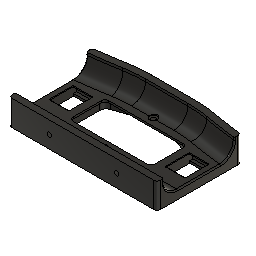
Filtered Mains Braket (Autodesk Fusion 360 design; units mm, degrees)
Autodesk Fusion 360 part; units mm, degrees
sketch "Mains Cutout" plane through (0, 0, 0) normal (0, 0, 1) x (1, 0, 0)
  line L0 (0, 25.5) -> (0, -25.5) construction
  line L1 (-33.15, 14.516) -> (33.15, -14.516) construction
  line L2 (33.15, 14.516) -> (-33.15, -14.516) construction
  line L3 (-33.15, 14.516) -> (33.15, 14.516) construction
  line L4 (33.15, 14.516) -> (33.15, -14.516) construction
  line L5 (33.15, -14.516) -> (-33.15, -14.516) construction
  line L6 (-33.15, -10.9343) -> (-33.15, 14.516) construction
  line L7 (29.7587, -15.6684) -> (1.6087, -25.2341)
  line L8 (-29.7587, -15.6684) -> (-1.6087, -25.2341)
  line L9 (-29.7587, 15.6684) -> (-1.6087, 25.2341)
  line L10 (29.7587, 15.6684) -> (1.6087, 25.2341)
  arc A0 (1.6087, 25.2341) -> (-1.6087, 25.2341) centre (0, 20.5) ccw
  arc A1 (-1.6087, -25.2341) -> (1.6087, -25.2341) centre (0, -20.5) ccw
  line L11 (33.15, 10.9343) -> (33.15, -10.9343) construction
  line L12 (-33.15, -14.516) -> (-33.15, 10.9343) construction
  circle A2 centre (0, 20) radius 1.65
  circle A3 centre (0, -20) radius 1.65
  line L13 (0, 20) -> (0, -20) construction
  circle A4 centre (0, 20) radius 3
  circle A5 centre (0, -20) radius 3
  line L14 (-29.2, 14.1) -> (29.2, 14.1)
  line L15 (32.2, 11.1) -> (32.2, -11.1)
  line L16 (29.2, -14.1) -> (-29.2, -14.1)
  line L17 (-32.2, -11.1) -> (-32.2, 11.1)
  arc A6 (32.2, 11.1) -> (29.2, 14.1) centre (29.2, 11.1) ccw
  arc A7 (29.2, -14.1) -> (32.2, -11.1) centre (29.2, -11.1) ccw
  arc A8 (-32.2, -11.1) -> (-29.2, -14.1) centre (-29.2, -11.1) ccw
  line L18 (29.2, 14.1) -> (32.2, 14.1) construction
  line L19 (32.2, 11.1) -> (32.2, 14.1) construction
  line L20 (32.2, -11.1) -> (32.2, -14.1) construction
  line L21 (29.2, -14.1) -> (32.2, -14.1) construction
  line L22 (-29.2, -14.1) -> (-32.2, -14.1) construction
  line L23 (-32.2, -11.1) -> (-32.2, -14.1) construction
  arc A9 (-29.2, 14.1) -> (-32.2, 11.1) centre (-29.2, 11.1) ccw
  line L24 (-29.2, 14.1) -> (-32.2, 14.1) construction
  line L25 (-32.2, 11.1) -> (-32.2, 14.1) construction
  arc A10 (-29.7587, 15.6684) -> (-33.15, 10.9343) centre (-28.15, 10.9343) ccw
  line L26 (-29.7587, 15.6684) -> (-33.15, 14.516) construction
  arc A11 (-33.15, -10.9343) -> (-29.7587, -15.6684) centre (-28.15, -10.9343) ccw
  line L27 (-29.7587, -15.6684) -> (-33.15, -14.516) construction
  line L28 (-33.15, 10.9343) -> (-33.15, -10.9343)
  arc A12 (33.15, 10.9343) -> (29.7587, 15.6684) centre (28.15, 10.9343) ccw
  arc A13 (29.7587, -15.6684) -> (33.15, -10.9343) centre (28.15, -10.9343) ccw
  line L29 (29.7587, -15.6684) -> (33.15, -14.516) construction
  line L30 (29.7587, 15.6684) -> (33.15, 14.516) construction
  line L31 (33.15, 10.9343) -> (33.15, -10.9343)
  arc A14 (2.2522, 27.1278) -> (-2.2522, 27.1278) centre (0, 20.5) ccw
  line L32 (-30.4022, 17.562) -> (-2.2522, 27.1278)
  arc A15 (-30.4022, 17.562) -> (-35.15, 10.9343) centre (-28.15, 10.9343) ccw
  line L33 (-35.15, 10.9343) -> (-35.15, -10.9343)
  arc A16 (-35.15, -10.9343) -> (-30.4022, -17.562) centre (-28.15, -10.9343) ccw
  line L34 (-30.4022, -17.562) -> (-2.2522, -27.1278)
  arc A17 (-2.2522, -27.1278) -> (2.2522, -27.1278) centre (0, -20.5) ccw
  line L35 (30.4022, -17.562) -> (2.2522, -27.1278)
  arc A18 (30.4022, -17.562) -> (35.15, -10.9343) centre (28.15, -10.9343) ccw
  line L36 (35.15, 10.9343) -> (35.15, -10.9343)
  arc A19 (35.15, 10.9343) -> (30.4022, 17.562) centre (28.15, 10.9343) ccw
  line L37 (30.4022, 17.562) -> (2.2522, 27.1278)
  dimension "d6" = 3
  dimension "d7" = 3
  dimension "d8" = 3
  dimension "d10" = 40
  dimension "d11" = 28.2
  dimension "d12" = 51
  dimension "d13" = 5
  dimension "d14" = 5
  dimension "d15" = 64.4
  dimension "d16" = 66.3
  dimension "d17" = 3
  dimension "d18" = 5
  dimension "d19" = 5
  dimension "d20" = 5
  dimension "d21" = 5
  dimension "d22" = 3.3
  dimension "d23" = 6
  dimension "d24" = 3.3
  dimension "d25" = 6
  dimension "d26" = -2
  constraint vertical L0
  constraint midpoint origin L0
  constraint midpoint origin L2
  constraint midpoint origin L1
  constraint vertical L4
  constraint horizontal L5
  constraint vertical L6
  constraint coincident L2.start L3.end
  constraint coincident L0 A0.centre
  constraint coincident L0.start A0
  constraint coincident L0 A1.centre
  constraint coincident L0.end A1
  constraint tangent L7 A1
  constraint tangent L8 A1
  constraint tangent L9 A0
  constraint tangent L10 A0
  constraint coincident L2.end L6
  constraint coincident L2.start L4
  constraint perpendicular L3 L11
  constraint coincident L0 A2.centre
  constraint coincident L0 A3.centre
  constraint coincident A2.centre L13.start
  constraint coincident A3.centre L13.end
  constraint midpoint origin L13
  constraint concentric A3 A5
  constraint vertical L15
  constraint horizontal L16
  constraint vertical L17
  constraint tangent L14 A6
  constraint tangent L15 A6
  constraint tangent L15 A7
  constraint tangent L16 A7
  constraint tangent L16 A8
  constraint tangent L17 A8
  constraint coincident L2 L18.end
  constraint tangent A6 L18
  constraint coincident L1 L20.end
  constraint coincident L2 L22.end
  constraint tangent A8 L23
  constraint collinear L15 L19
  constraint collinear L15 L20
  constraint collinear L16 L21
  constraint horizontal L14
  constraint coincident L1 L24.end
  constraint tangent A9 L24
  constraint tangent L17 A9
  constraint collinear L17 L25
  constraint collinear L14 L24
  constraint coincident L1.start L9
  constraint tangent L9 A10
  constraint tangent L12 A10
  constraint coincident L1.start L3.start
  constraint coincident L2.end L8
  constraint tangent L6 A11
  constraint tangent L8 A11
  constraint coincident L2.end L5.end
  constraint coincident L2.start L10
  constraint coincident L2.start L11
  constraint tangent L10 A12
  constraint tangent L11 A12
  constraint coincident L1.end L7
  constraint tangent L7 A13
  constraint tangent L11 A13
  constraint collinear L7 L29
  constraint coincident L1.end L4.end
  constraint collinear L4 L11
  measures "d6" radius of A8
  measures "d7" radius of A7
  measures "d8" radius of A6
  measures "d10" distance of A2.centre A3.centre
  measures "d11" distance of L14 L16
  measures "d12" distance of L0.start L0.end
  measures "d13" radius of A0
  measures "d14" radius of A1
  measures "d15" distance of L15 L17
  measures "d16" distance of L4 L12
  measures "d17" radius of A9
  measures "d18" radius of A10
  measures "d19" radius of A11
  measures "d20" radius of A12
  measures "d21" radius of A13
  measures "d22" diameter of A2
  measures "d23" diameter of A4
  measures "d24" diameter of A3
  measures "d25" diameter of A5
extrude "Extrude1" add sketch "Mains Cutout" along normal blind 4 contours A14 L32 A15 L33 A16 L34 A17 L35 A18 L36 A19 L37 makes body 1
extrude "Extrude2" add sketch "Mains Cutout" along normal blind 2 contours L7 L8 L9 L10 A0 A1 A10 A11 L28 A12 A13 L31 | A2 | A3 | A4 | A5 bodies 1
extrude "Extrude3" cut sketch "Mains Cutout" along normal blind 1 contours A2 | A3 | A4 | A5 bodies 1
extrude "Extrude4" cut sketch "Mains Cutout" along normal blind 5 from surface at 1.2 contours A2 | A3 bodies 1
sketch "Body" plane through (0, 0, 0) normal (0, 0, 1) x (1, 0, 0)
  line L0 (-25.8441, 35.5) -> (0, 35.5)
  line L1 (0, 35.5) -> (0, -35.5)
  line L2 (0, -35.5) -> (-58.5, -35.5)
  line L3 (-58.5, -35.5) -> (-58.5, 30.4101)
  arc A0 (-58.5, 30.4101) -> (-25.8441, 35.5) centre (-108.5, 458.5) ccw
  arc A1 (-58.5, 25.3765) -> (-25.3616, 30.5) centre (-108.5, 458.5) ccw
  line L4 (-25.3616, 30.5) -> (0, 30.5)
  line L5 (0, -30.5) -> (-58.5, -30.5)
  dimension "d36" = 58.5
  dimension "d38" = 50
  dimension "d39" = 494
  dimension "d40" = 862
  dimension "d41" = 71
  dimension "d43" = 5
  dimension "d44" = 5
  dimension "d45" = 5
  constraint horizontal L0
  constraint vertical L1
  constraint horizontal L2
  constraint vertical L3
  constraint coincident origin L1
  constraint midpoint L1 origin
  constraint concentric A0 A1
  constraint parallel L0 L4
  constraint coincident L3 A1.start
  constraint coincident L1 L5.start
  constraint coincident L3 L5.end
  constraint perpendicular L3 L5
  measures "d36" distance of L1.end L2.end
  measures "d38" horizontal distance of L2.end A0.centre
  measures "d39" vertical distance of L2.end A0.centre
  measures "d40" diameter of A0
  measures "d41" distance of L0 L2
  measures "d43" distance of A0 A1
  measures "d44" distance of L0 L4
  measures "d45" distance of L2 L5
extrude "Extrude5" add sketch "Body" along normal blind 7 separate body makes body 2
extrude "Extrude6" add sketch "Body" along normal blind 20 contours L0 L1 L3 A0 A1 L4 | L1 L2 L3 L5 bodies 2
sketch "Keystone" plane through (0, 0, 0) normal (1, 0, 0) x (0, 1, 0)
  line L0 (25.3765, 7) -> (-30.5, 7) construction
  line L1 (-35.5, 0) -> (30.4101, 0) construction
  line L2 (10.325, -9.0063) -> (-10.325, -9.0063)
  line L3 (-10.325, -10.7563) -> (-12.375, -10.7563)
  line L4 (-12.375, -10.7563) -> (-12.375, -11.8863)
  line L5 (-12.375, -11.8863) -> (-8.525, -15.7363)
  line L6 (-8.525, -15.7363) -> (-8.525, -16.0063)
  line L7 (10.325, -16.0063) -> (10.325, -15.1063)
  line L8 (10.325, -15.1063) -> (12.825, -12.6063)
  line L9 (12.825, -12.6063) -> (12.825, -10.7563)
  line L10 (12.825, -10.7563) -> (10.325, -10.7563)
  line L11 (10.325, -9.0063) -> (10.325, -10.7563)
  line L12 (-10.325, -9.0063) -> (-10.325, -10.7563)
  line L13 (10.325, -16.0063) -> (-8.525, -16.0063)
  line L14 (0, -9.0063) -> (0, 0) construction
  line L15 (10.325, 0) -> (10.325, 1.75)
  line L16 (10.325, 1.75) -> (12.825, 1.75)
  line L17 (12.825, 1.75) -> (12.825, 3.6)
  line L18 (12.825, 3.6) -> (10.325, 6.1)
  line L19 (10.325, 6.1) -> (10.325, 7)
  line L20 (-10.325, 0) -> (-10.325, 1.75)
  line L21 (-10.325, 1.75) -> (-12.375, 1.75)
  line L22 (-12.375, 1.75) -> (-12.375, 2.88)
  line L23 (-12.375, 2.88) -> (-8.525, 6.73)
  line L24 (-8.525, 6.73) -> (-8.525, 7)
  line L25 (10.325, 7) -> (-8.525, 7)
  line L26 (-10.325, 0) -> (10.325, 0)
  dimension "d78" = 20.65
  dimension "d79" = 1.75
  dimension "d80" = 3.85
  dimension "d81" = 0.27
  dimension "d82" = 18.85
  dimension "d83" = 1.85
  dimension "d84" = 1.75
  dimension "d85" = 2.5
  dimension "d86" = 135
  dimension "d87" = 135
  dimension "d96" = 0.9
  dimension "d97" = 135
  dimension "d98" = 135
  dimension "d99" = 0.27
  dimension "d100" = 1.75
  dimension "d101" = 2.5
  dimension "d102" = 1.85
  dimension "d103" = 18.85
  dimension "d104" = 20.65
  dimension "d105" = 1.75
  dimension "d106" = 3.85
  constraint parallel L0 L3
  constraint perpendicular L0 L4
  constraint perpendicular L1 L6
  constraint perpendicular L1 L7
  constraint perpendicular L1 L9
  constraint perpendicular L9 L10
  constraint perpendicular L3 L12
  constraint perpendicular L2 L11
  constraint collinear L7 L11
  constraint coincident L14.end origin
  constraint midpoint L2 L14.start
  constraint perpendicular L2 L14
  constraint coincident L1 L15.start
  constraint perpendicular L1 L15
  constraint perpendicular L15 L16
  constraint perpendicular L1 L17
  constraint coincident L0 L19.end
  constraint perpendicular L0 L19
  constraint coincident L1 L20.start
  constraint perpendicular L0 L20
  constraint perpendicular L15 L21
  constraint perpendicular L0 L22
  constraint coincident L0 L24.end
  constraint perpendicular L0 L24
  constraint collinear L15 L19
  constraint midpoint L14.end L26
  measures "d78" distance of L2.start L2.end
  measures "d79" distance of L2.end L3.start
  measures "d80" horizontal distance of L4.end L5.end
  measures "d81" distance of L5.end L6.end
  measures "d82" distance of L6.end L7.start
  measures "d83" distance of L8.end L9.end
  measures "d84" vertical distance of L2.start L10.end
  measures "d85" distance of L9.end L10.end
  measures "d86" angle of L4 L5
  measures "d87" angle of L8 L9
  measures "d96" distance of L7.start L7.end
  measures "d97" angle of L17 L18
  measures "d98" angle of L22 L23
  measures "d99" distance of L23.end L24.end
  measures "d100" distance of L15.start L15.end
  measures "d101" distance of L15.end L16.end
  measures "d102" distance of L16.end L17.end
  measures "d103" distance of L19.end L24.end
  measures "d104" distance of L15.start L20.start
  measures "d105" distance of L20.start L20.end
  measures "d106" horizontal distance of L22.end L23.end
extrude "Extrude12" cut sketch "Keystone" against normal blind 14.9 from surface at -38.36 contours L15 L16 L17 L18 L19 L20 L21 L22 L23 L24 L25 L26 bodies 2
chamfer "Chamfer1" distance 0.4 angle 45 2 edges at (-53.26, 0.9, 7) (-38.36, 0.9, 7) on bodies 2
fillet "Fillet1" radius 95 1 edges at (-25.3616, 30.5, 13.5) on bodies 2
fillet "Fillet2" radius 100 1 edges at (-25.8441, 35.5, 10) on bodies 2
fillet "Fillet3" radius 11 3 edges at (-8.337, 30.5, 7) (-24.9194, 30.1415, 7) (-45.774, 27.0357, 7) on bodies 2
fillet "Fillet4" radius 11 1 edges at (-29.25, -30.5, 7) on bodies 2
fillet "Fillet5" radius 1 5 edges at (-58.5, 25.3765, 19) (-58.5, 22.1224, 10.2109) (-58.5, -2.5974, 7) (-58.5, -27.2782, 10.2218) (-58.5, -30.5, 19) on bodies 2
fillet "Fillet6" radius 2.5 2 edges at (-58.5, -35.5, 10) (-58.5, 30.4101, 10) on bodies 2
sketch "Mounting Holes" plane through (0, -35.5, 0) normal (0, -1, 0) x (1, 0, 0)
  line L0 (-56, 20) -> (-56, 0)
  line L1 (-56, 0) -> (0, 0)
  line L2 (0, 0) -> (0, 20)
  line L3 (0, 20) -> (-56, 20)
  circle A0 centre (-26.5, 10) radius 1.7
  line L4 (-58.5, 20) -> (-58.5, 0)
  circle A1 centre (-26.5, 10) radius 3
  dimension "d73" = 3.4
  dimension "d74" = 32
  dimension "d75" = 10
  dimension "d92" = 6
  constraint concentric A0 A1
  measures "d73" diameter of A0
  measures "d74" distance of A0.centre L4
  measures "d75" vertical distance of L1.end A0.centre
  measures "d92" diameter of A1
extrude "Extrude11" cut sketch "Mounting Holes" against normal blind 29 contours A0 bodies 2
extrude "Extrude13" cut sketch "Mounting Holes" against normal blind 16.5 from surface at -3 contours A1 bodies 2
mirror "Mirror1" about plane through (0, 0, 0) normal (1, 0, 0) of bodies 2 merged
extrude "Extrude7" cut sketch "Mains Cutout" along normal through all contours L14 L15 L16 L17 A6 A7 A8 A9 bodies 2
extrude "Extrude8" cut sketch "Mains Cutout" along normal up to surface (5.5 mm away) contours L7 L8 L9 L10 A0 A1 A10 A11 L28 A12 A13 L31 | A2 | A3 | A4 | A5 bodies 2
extrude "Extrude9" cut sketch "Mains Cutout" along normal through all and the other way blind 0.5 from surface at 7 contours A2 | A3 | A4 | A5 bodies 2
extrude "Extrude10" cut sketch "Mains Cutout" along normal up to surface (6.3 mm away) contours A2 | A3 bodies 2
hidden bodies 1
